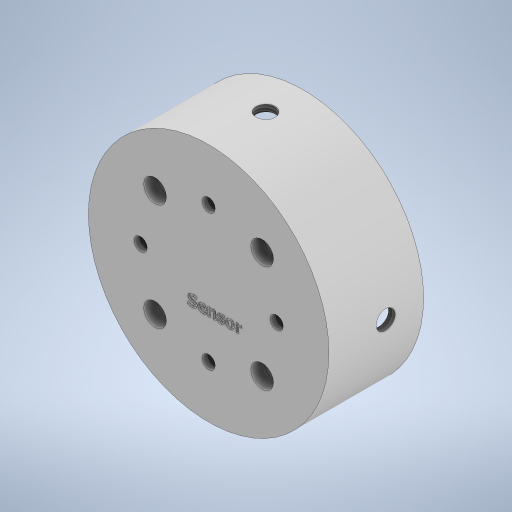
# Autodesk Inventor part: adaptor_sensor_spine
Saved by Autodesk Inventor 2024 (Build 280153000, 153)
## iProperties
Created: 2024-05-24
Part Number: adaptor_sensor_spine
Material: Generic
Document SubType Name: Modeling
Designer: maint
Density: 1 g/cm^3
Appearance: Default
Author: maint
Autodesk Inventor part; units mm, degrees
ref_plane "YZ Plane" through (0, 0, 0) normal (1, 0, 0) x (0, 1, 0)
sketch "Sketch1" plane through (0, 0, 0) normal (0, 0, 1) x (1, 0, 0)
  line L0 (40, -40) -> (-40, -40)
  line L1 (-40, -40) -> (-40, 40)
  line L2 (-40, 40) -> (40, 40)
  line L3 (40, 40) -> (40, -40)
  line L4 (40, -40) -> (-40, 40) construction
  line L5 (-40, -40) -> (40, 40) construction
  circle A0 centre (0, 0) radius 63.5
  dimension "d0" = 80
  dimension "d72" = 127
  constraints: 12 end point, 2 midpoint, 2 parallel, 2 perpendicular, 1 centre point, 1 coincident, 1 horizontal
  measures "d0" distance of L1.end L2.end
  measures "d72" diameter of A0
extrude "Extrusion1" add sketch "Sketch1" along normal blind 10 contours L0 L1 L2 L3 | A0
sketch "Sketch2" plane through (0, 0, 0) normal (0, 0, -1) x (-1, 0, 0)
  arc A0 (40, 37) -> (37, 40) centre (37, 37) ccw
  line L0 (28.2843, -28.2843) -> (-28.2843, -28.2843)
  line L1 (-28.2843, -28.2843) -> (-28.2843, 28.2843)
  line L2 (-28.2843, 28.2843) -> (28.2843, 28.2843)
  line L3 (28.2843, 28.2843) -> (28.2843, -28.2843)
  line L4 (28.2843, -28.2843) -> (-28.2843, 28.2843) construction
  line L5 (-28.2843, -28.2843) -> (28.2843, 28.2843) construction
  circle A1 centre (-28.2843, 28.2843) radius 4.75
  circle A2 centre (28.2843, 28.2843) radius 4.75
  circle A3 centre (28.2843, -28.2843) radius 4.75
  circle A4 centre (-28.2843, -28.2843) radius 4.75
  circle A5 centre (0, 0) radius 40
  point P0 (39.1213, 39.1213)
  dimension "d63" = 12
  dimension "d129" = 80
  dimension "d33" = 9.5
  constraints: 12 end point, 5 centre point, 5 coincident, 3 equal radius, 3 point on circle, 2 midpoint, 2 parallel, 2 perpendicular, 1 horizontal, 3 other
  measures "d33" diameter of A2
hole "Hole3" at (28.2843, -28.2843, 0) at (28.2843, 28.2843, 0) at (-28.2843, 28.2843, 0) at (-28.2843, -28.2843, 0) direction (0, 0, 1) diameter 6.6 end through all
sketch "Sketch10" plane through (0, 0, 10) normal (0, 0, 1) x (1, 0, 0)
  circle A0 centre (28.2843, 28.2843) radius 3.3 projected
  circle A1 centre (28.2843, 28.2843) radius 6
  circle A2 centre (-28.2843, 28.2843) radius 3.3 projected
  circle A3 centre (-28.2843, 28.2843) radius 6
  circle A4 centre (0, 0) radius 40
  line L0 (28.2843, 28.2843) -> (-28.2843, 28.2843)
  line L1 (-28.2843, 28.2843) -> (-28.2843, -28.2843)
  line L2 (-28.2843, -28.2843) -> (28.2843, -28.2843)
  line L3 (28.2843, -28.2843) -> (28.2843, 28.2843)
  circle A5 centre (-28.2843, -28.2843) radius 3.3 projected
  circle A6 centre (-28.2843, -28.2843) radius 6
  circle A7 centre (28.2843, -28.2843) radius 6
  dimension "d63" = 12
  dimension "d127" = 80
  constraints: 8 end point, 5 centre point, 5 coincident, 3 equal radius, 2 parallel, 1 horizontal, 1 perpendicular
  measures "d63" diameter of A1
  measures "d127" diameter of A4
sketch "Sketch11" plane through (-1.9817, 2.6504, 0) normal (0, 0, -1) x (-1, 0, 0)
  line L0 (-12.9782, -14.2221) -> (9.0418, -14.2221) construction
  line L1 (9.0418, -14.2221) -> (9.0418, -6.8756) construction
  line L2 (9.0418, -6.8756) -> (-12.9782, -6.8756) construction
  line L3 (-12.9782, -6.8756) -> (-12.9782, -14.2221) construction
  spline S0 degree 2 poles (-10.4621, -20.5396) (-11.164, -20.5396) (-12.2219, -20.2677) (-12.6767, -20.07) knots 0 0 0 1 2 2 2
  line L4 (-12.6767, -20.07) -> (-12.6767, -18.6166)
  line L5 (-12.6767, -18.6166) -> (-12.5383, -18.6166)
  spline S1 degree 2 poles (-12.5383, -18.6166) (-12.0785, -19.0072) (-10.9762, -19.4273) (-10.4571, -19.4273) knots 0 0 0 1 2 2 2
  spline S2 degree 2 poles (-10.4571, -19.4273) (-10.3237, -19.4273) (-9.8936, -19.368) (-9.7651, -19.3087) knots 0 0 0 1 2 2 2
  spline S3 degree 2 poles (-9.7651, -19.3087) (-9.6069, -19.2395) (-9.3845, -18.9874) (-9.3845, -18.7847) knots 0 0 0 1 2 2 2
  spline S4 degree 2 poles (-9.3845, -18.7847) (-9.3845, -18.5524) (-9.7453, -18.2657) (-9.9925, -18.2014) knots 0 0 0 1 2 2 2
  spline S5 degree 2 poles (-9.9925, -18.2014) (-10.3039, -18.1174) (-11.0108, -17.974) (-11.3222, -17.8653) knots 0 0 0 1 2 2 2
  spline S6 degree 2 poles (-11.3222, -17.8653) (-12.0291, -17.6181) (-12.6421, -16.7728) (-12.6421, -16.1401) knots 0 0 0 1 2 2 2
  spline S7 degree 2 poles (-12.6421, -16.1401) (-12.6421, -15.2849) (-11.1937, -14.2221) (-10.1062, -14.2221) knots 0 0 0 1 2 2 2
  spline S8 degree 2 poles (-10.1062, -14.2221) (-9.5624, -14.2221) (-8.4848, -14.4445) (-8.0597, -14.6324) knots 0 0 0 1 2 2 2
  line L6 (-8.0597, -14.6324) -> (-8.0597, -16.0264)
  line L7 (-8.0597, -16.0264) -> (-8.1931, -16.0264)
  spline S9 degree 2 poles (-8.1931, -16.0264) (-8.5342, -15.7347) (-9.513, -15.3343) (-10.0271, -15.3343) knots 0 0 0 1 2 2 2
  spline S10 degree 2 poles (-10.0271, -15.3343) (-10.2298, -15.3343) (-10.5461, -15.3936) (-10.7241, -15.4727) knots 0 0 0 1 2 2 2
  spline S11 degree 2 poles (-10.7241, -15.4727) (-10.8674, -15.537) (-11.0751, -15.794) (-11.0751, -15.9522) knots 0 0 0 1 2 2 2
  spline S12 degree 2 poles (-11.0751, -15.9522) (-11.0751, -16.1895) (-10.7439, -16.4614) (-10.2693, -16.5701) knots 0 0 0 1 2 2 2
  spline S13 degree 2 poles (-10.2693, -16.5701) (-9.9628, -16.6393) (-9.3943, -16.7728) (-9.0681, -16.8865) knots 0 0 0 1 2 2 2
  spline S14 degree 2 poles (-9.0681, -16.8865) (-8.4353, -17.1188) (-7.8174, -17.89) (-7.8174, -18.5227) knots 0 0 0 1 2 2 2
  spline S15 degree 2 poles (-7.8174, -18.5227) (-7.8174, -19.4323) (-9.246, -20.5396) (-10.4621, -20.5396) knots 0 0 0 1 2 2 2
  spline S16 degree 2 poles (-2.3403, -16.2538) (-2.3403, -16.6789) (-2.6122, -17.45) (-2.8643, -17.7071) knots 0 0 0 1 2 2 2
  spline S17 degree 2 poles (-2.8643, -17.7071) (-3.0175, -17.8702) (-3.3932, -18.1371) (-3.6157, -18.2311) knots 0 0 0 1 2 2 2
  spline S18 degree 2 poles (-3.6157, -18.2311) (-3.843, -18.325) (-4.372, -18.4337) (-4.6982, -18.4337) knots 0 0 0 1 2 2 2
  line L8 (-4.6982, -18.4337) -> (-5.499, -18.4337)
  line L9 (-5.499, -18.4337) -> (-5.499, -20.4308)
  line L10 (-5.499, -20.4308) -> (-7.0315, -20.4308)
  line L11 (-7.0315, -20.4308) -> (-7.0315, -14.3308)
  line L12 (-7.0315, -14.3308) -> (-4.6636, -14.3308)
  spline S19 degree 2 poles (-4.6636, -14.3308) (-4.1396, -14.3308) (-3.3734, -14.5236) (-3.062, -14.7312) knots 0 0 0 1 2 2 2
  spline S20 degree 2 poles (-3.062, -14.7312) (-2.716, -14.9636) (-2.3403, -15.7248) (-2.3403, -16.2538) knots 0 0 0 1 2 2 2
  spline S21 degree 2 poles (-3.9122, -16.2933) (-3.9122, -16.0313) (-4.1594, -15.6606) (-4.3275, -15.5914) knots 0 0 0 1 2 2 2
  spline S22 degree 2 poles (-4.3275, -15.5914) (-4.545, -15.4974) (-4.9404, -15.4678) (-5.2815, -15.4678) knots 0 0 0 1 2 2 2
  line L13 (-5.2815, -15.4678) -> (-5.499, -15.4678)
  line L14 (-5.499, -15.4678) -> (-5.499, -17.2968)
  line L15 (-5.499, -17.2968) -> (-5.3903, -17.2968)
  spline S23 degree 2 poles (-5.3903, -17.2968) (-5.1777, -17.2968) (-4.7922, -17.2869) (-4.6488, -17.2622) knots 0 0 0 1 2 2 2
  spline S24 degree 2 poles (-4.6488, -17.2622) (-4.5252, -17.2424) (-4.2533, -17.1238) (-4.1792, -17.0496) knots 0 0 0 1 2 2 2
  spline S25 degree 2 poles (-4.1792, -17.0496) (-4.021, -16.9013) (-3.9122, -16.5701) (-3.9122, -16.2933) knots 0 0 0 1 2 2 2
  line L16 (1.5155, -20.4308) -> (-1.7669, -20.4308)
  line L17 (-1.7669, -20.4308) -> (-1.7669, -19.368)
  line L18 (-1.7669, -19.368) -> (-0.8919, -19.368)
  line L19 (-0.8919, -19.368) -> (-0.8919, -15.3936)
  line L20 (-0.8919, -15.3936) -> (-1.7669, -15.3936)
  line L21 (-1.7669, -15.3936) -> (-1.7669, -14.3308)
  line L22 (-1.7669, -14.3308) -> (1.5155, -14.3308)
  line L23 (1.5155, -14.3308) -> (1.5155, -15.3936)
  line L24 (1.5155, -15.3936) -> (0.6405, -15.3936)
  line L25 (0.6405, -15.3936) -> (0.6405, -19.368)
  line L26 (0.6405, -19.368) -> (1.5155, -19.368)
  line L27 (1.5155, -19.368) -> (1.5155, -20.4308)
  line L28 (7.7588, -20.4308) -> (6.2857, -20.4308)
  line L29 (6.2857, -20.4308) -> (3.9327, -16.1796)
  line L30 (3.9327, -16.1796) -> (3.9327, -20.4308)
  line L31 (3.9327, -20.4308) -> (2.5338, -20.4308)
  line L32 (2.5338, -20.4308) -> (2.5338, -14.3308)
  line L33 (2.5338, -14.3308) -> (4.4122, -14.3308)
  line L34 (4.4122, -14.3308) -> (6.3599, -17.8257)
  line L35 (6.3599, -17.8257) -> (6.3599, -14.3308)
  line L36 (6.3599, -14.3308) -> (7.7588, -14.3308)
  line L37 (7.7588, -14.3308) -> (7.7588, -20.4308)
  line L38 (8.9996, -20.4308) -> (8.9996, -14.3308)
  line L39 (8.9996, -14.3308) -> (13.1223, -14.3308)
  line L40 (13.1223, -14.3308) -> (13.1223, -15.4925)
  line L41 (13.1223, -15.4925) -> (10.5221, -15.4925)
  line L42 (10.5221, -15.4925) -> (10.5221, -16.5652)
  line L43 (10.5221, -16.5652) -> (12.9196, -16.5652)
  line L44 (12.9196, -16.5652) -> (12.9196, -17.7268)
  line L45 (12.9196, -17.7268) -> (10.5221, -17.7268)
  line L46 (10.5221, -17.7268) -> (10.5221, -19.2692)
  line L47 (10.5221, -19.2692) -> (13.1223, -19.2692)
  line L48 (13.1223, -19.2692) -> (13.1223, -20.4308)
  line L49 (13.1223, -20.4308) -> (8.9996, -20.4308)
  point P0 (0, 0)
  constraints: 2 other
extrude "Extrusion5" cut sketch "Sketch11" against normal blind 1
sketch "Sketch12" plane through (-4.4722, 1.3995, 10) normal (0, 0, 1) x (1, 0, 0)
  line L0 (-6.7643, -10.3972) -> (19.0988, -10.3972) construction
  line L1 (19.0988, -10.3972) -> (19.0988, -6.1489) construction
  line L2 (19.0988, -6.1489) -> (-6.7643, -6.1489) construction
  line L3 (-6.7643, -6.1489) -> (-6.7643, -10.3972) construction
  spline S0 degree 2 poles (-4.2481, -16.7147) (-4.9501, -16.7147) (-6.0079, -16.4428) (-6.4627, -16.2451) knots 0 0 0 1 2 2 2
  line L4 (-6.4627, -16.2451) -> (-6.4627, -14.7918)
  line L5 (-6.4627, -14.7918) -> (-6.3243, -14.7918)
  spline S1 degree 2 poles (-6.3243, -14.7918) (-5.8646, -15.1823) (-4.7622, -15.6025) (-4.2432, -15.6025) knots 0 0 0 1 2 2 2
  spline S2 degree 2 poles (-4.2432, -15.6025) (-4.1097, -15.6025) (-3.6797, -15.5432) (-3.5511, -15.4838) knots 0 0 0 1 2 2 2
  spline S3 degree 2 poles (-3.5511, -15.4838) (-3.3929, -15.4146) (-3.1705, -15.1625) (-3.1705, -14.9599) knots 0 0 0 1 2 2 2
  spline S4 degree 2 poles (-3.1705, -14.9599) (-3.1705, -14.7275) (-3.5314, -14.4408) (-3.7785, -14.3765) knots 0 0 0 1 2 2 2
  spline S5 degree 2 poles (-3.7785, -14.3765) (-4.0899, -14.2925) (-4.7968, -14.1492) (-5.1083, -14.0404) knots 0 0 0 1 2 2 2
  spline S6 degree 2 poles (-5.1083, -14.0404) (-5.8152, -13.7932) (-6.4281, -12.9479) (-6.4281, -12.3152) knots 0 0 0 1 2 2 2
  spline S7 degree 2 poles (-6.4281, -12.3152) (-6.4281, -11.46) (-4.9797, -10.3972) (-3.8922, -10.3972) knots 0 0 0 1 2 2 2
  spline S8 degree 2 poles (-3.8922, -10.3972) (-3.3485, -10.3972) (-2.2708, -10.6197) (-1.8457, -10.8075) knots 0 0 0 1 2 2 2
  line L6 (-1.8457, -10.8075) -> (-1.8457, -12.2015)
  line L7 (-1.8457, -12.2015) -> (-1.9792, -12.2015)
  spline S9 degree 2 poles (-1.9792, -12.2015) (-2.3203, -11.9099) (-3.299, -11.5094) (-3.8131, -11.5094) knots 0 0 0 1 2 2 2
  spline S10 degree 2 poles (-3.8131, -11.5094) (-4.0158, -11.5094) (-4.3322, -11.5688) (-4.5101, -11.6479) knots 0 0 0 1 2 2 2
  spline S11 degree 2 poles (-4.5101, -11.6479) (-4.6535, -11.7121) (-4.8611, -11.9692) (-4.8611, -12.1274) knots 0 0 0 1 2 2 2
  spline S12 degree 2 poles (-4.8611, -12.1274) (-4.8611, -12.3646) (-4.5299, -12.6365) (-4.0553, -12.7453) knots 0 0 0 1 2 2 2
  spline S13 degree 2 poles (-4.0553, -12.7453) (-3.7489, -12.8145) (-3.1804, -12.9479) (-2.8541, -13.0616) knots 0 0 0 1 2 2 2
  spline S14 degree 2 poles (-2.8541, -13.0616) (-2.2214, -13.294) (-1.6035, -14.0651) (-1.6035, -14.6979) knots 0 0 0 1 2 2 2
  spline S15 degree 2 poles (-1.6035, -14.6979) (-1.6035, -15.6074) (-3.0321, -16.7147) (-4.2481, -16.7147) knots 0 0 0 1 2 2 2
  spline S16 degree 2 poles (1.4564, -16.7295) (0.1514, -16.7295) (-1.2377, -15.4838) (-1.2377, -14.3321) knots 0 0 0 1 2 2 2
  spline S17 degree 2 poles (-1.2377, -14.3321) (-1.2377, -13.205) (0.0575, -11.8604) (1.2241, -11.8604) knots 0 0 0 1 2 2 2
  spline S18 degree 2 poles (1.2241, -11.8604) (2.277, -11.8604) (3.3447, -13.0023) (3.3447, -14.0602) knots 0 0 0 1 2 2 2
  line L8 (3.3447, -14.0602) -> (3.3447, -14.5792)
  line L9 (3.3447, -14.5792) -> (0.1959, -14.5792)
  spline S19 degree 2 poles (0.1959, -14.5792) (0.2156, -14.9005) (0.448, -15.3257) (0.6358, -15.4542) knots 0 0 0 1 2 2 2
  spline S20 degree 2 poles (0.6358, -15.4542) (0.8187, -15.5827) (1.3131, -15.6915) (1.6047, -15.6915) knots 0 0 0 1 2 2 2
  spline S21 degree 2 poles (1.6047, -15.6915) (1.8519, -15.6915) (2.3363, -15.5827) (2.539, -15.4888) knots 0 0 0 1 2 2 2
  spline S22 degree 2 poles (2.539, -15.4888) (2.7169, -15.4146) (3.0135, -15.2317) (3.1075, -15.1625) knots 0 0 0 1 2 2 2
  line L10 (3.1075, -15.1625) -> (3.2607, -15.1625)
  line L11 (3.2607, -15.1625) -> (3.2607, -16.3489)
  spline S23 degree 2 poles (3.2607, -16.3489) (3.0827, -16.4181) (2.796, -16.5368) (2.539, -16.5961) knots 0 0 0 1 2 2 2
  spline S24 degree 2 poles (2.539, -16.5961) (2.3066, -16.6603) (1.8123, -16.7295) (1.4564, -16.7295) knots 0 0 0 1 2 2 2
  spline S25 degree 2 poles (1.931, -13.7141) (1.9211, -13.2594) (1.5207, -12.7799) (1.1104, -12.7799) knots 0 0 0 1 2 2 2
  spline S26 degree 2 poles (1.1104, -12.7799) (0.6902, -12.7799) (0.2156, -13.2841) (0.1909, -13.7141) knots 0 0 0 1 2 2 2
  line L12 (0.1909, -13.7141) -> (1.931, -13.7141)
  line L13 (8.3869, -16.606) -> (6.9434, -16.606)
  line L14 (6.9434, -16.606) -> (6.9434, -14.3271)
  spline S27 degree 2 poles (6.9434, -14.3271) (6.9434, -14.0453) (6.8989, -13.4917) (6.8396, -13.3632) knots 0 0 0 1 2 2 2
  spline S28 degree 2 poles (6.8396, -13.3632) (6.7655, -13.205) (6.4887, -13.0715) (6.2514, -13.0715) knots 0 0 0 1 2 2 2
  spline S29 degree 2 poles (6.2514, -13.0715) (6.0784, -13.0715) (5.7175, -13.205) (5.5148, -13.3483) knots 0 0 0 1 2 2 2
  line L15 (5.5148, -13.3483) -> (5.5148, -16.606)
  line L16 (5.5148, -16.606) -> (4.0813, -16.606)
  line L17 (4.0813, -16.606) -> (4.0813, -12.0038)
  line L18 (4.0813, -12.0038) -> (5.5148, -12.0038)
  line L19 (5.5148, -12.0038) -> (5.5148, -12.5129)
  spline S30 degree 2 poles (5.5148, -12.5129) (5.8658, -12.2163) (6.5331, -11.8802) (6.9385, -11.8802) knots 0 0 0 1 2 2 2
  spline S31 degree 2 poles (6.9385, -11.8802) (7.6404, -11.8802) (8.3869, -12.77) (8.3869, -13.6103) knots 0 0 0 1 2 2 2
  line L20 (8.3869, -13.6103) -> (8.3869, -16.606)
  spline S32 degree 2 poles (10.8486, -16.7295) (10.3444, -16.7295) (9.4398, -16.5071) (9.1432, -16.3588) knots 0 0 0 1 2 2 2
  line L21 (9.1432, -16.3588) -> (9.1432, -15.1477)
  line L22 (9.1432, -15.1477) -> (9.2618, -15.1477)
  spline S33 degree 2 poles (9.2618, -15.1477) (9.3656, -15.2268) (9.6276, -15.4146) (9.86, -15.5184) knots 0 0 0 1 2 2 2
  spline S34 degree 2 poles (9.86, -15.5184) (10.0626, -15.6124) (10.5619, -15.7458) (10.8585, -15.7458) knots 0 0 0 1 2 2 2
  spline S35 degree 2 poles (10.8585, -15.7458) (11.1601, -15.7458) (11.6247, -15.558) (11.6247, -15.3553) knots 0 0 0 1 2 2 2
  spline S36 degree 2 poles (11.6247, -15.3553) (11.6247, -15.1971) (11.4122, -15.0291) (11.1057, -14.9599) knots 0 0 0 1 2 2 2
  spline S37 degree 2 poles (11.1057, -14.9599) (10.9425, -14.9154) (10.4433, -14.8214) (10.2505, -14.7621) knots 0 0 0 1 2 2 2
  spline S38 degree 2 poles (10.2505, -14.7621) (9.7067, -14.594) (9.163, -13.9366) (9.163, -13.3978) knots 0 0 0 1 2 2 2
  spline S39 degree 2 poles (9.163, -13.3978) (9.163, -13.0913) (9.4447, -12.5475) (9.7216, -12.335) knots 0 0 0 1 2 2 2
  spline S40 degree 2 poles (9.7216, -12.335) (9.9934, -12.1274) (10.7992, -11.8802) (11.3084, -11.8802) knots 0 0 0 1 2 2 2
  spline S41 degree 2 poles (11.3084, -11.8802) (11.7928, -11.8802) (12.6035, -12.073) (12.8803, -12.2064) knots 0 0 0 1 2 2 2
  line L23 (12.8803, -12.2064) -> (12.8803, -13.3731)
  line L24 (12.8803, -13.3731) -> (12.7666, -13.3731)
  spline S42 degree 2 poles (12.7666, -13.3731) (12.6925, -13.3137) (12.3712, -13.121) (12.2229, -13.0517) knots 0 0 0 1 2 2 2
  spline S43 degree 2 poles (12.2229, -13.0517) (12.04, -12.9727) (11.5951, -12.8639) (11.3627, -12.8639) knots 0 0 0 1 2 2 2
  spline S44 degree 2 poles (11.3627, -12.8639) (11.0513, -12.8639) (10.6212, -13.0765) (10.6212, -13.2495) knots 0 0 0 1 2 2 2
  spline S45 degree 2 poles (10.6212, -13.2495) (10.6212, -13.4077) (10.8338, -13.5856) (11.1897, -13.6746) knots 0 0 0 1 2 2 2
  spline S46 degree 2 poles (11.1897, -13.6746) (11.3726, -13.7191) (11.8521, -13.8031) (12.0746, -13.8773) knots 0 0 0 1 2 2 2
  spline S47 degree 2 poles (12.0746, -13.8773) (12.5689, -14.0355) (13.083, -14.6534) (13.083, -15.1675) knots 0 0 0 1 2 2 2
  spline S48 degree 2 poles (13.083, -15.1675) (13.083, -15.4888) (12.7814, -16.077) (12.4997, -16.2748) knots 0 0 0 1 2 2 2
  spline S49 degree 2 poles (12.4997, -16.2748) (12.208, -16.4923) (11.4072, -16.7295) (10.8486, -16.7295) knots 0 0 0 1 2 2 2
  spline S50 degree 2 poles (18.1795, -14.3073) (18.1795, -15.4443) (16.9387, -16.7493) (15.8067, -16.7493) knots 0 0 0 1 2 2 2
  spline S51 degree 2 poles (15.8067, -16.7493) (14.6797, -16.7493) (13.429, -15.4443) (13.429, -14.3073) knots 0 0 0 1 2 2 2
  spline S52 degree 2 poles (13.429, -14.3073) (13.429, -13.1605) (14.6797, -11.8604) (15.8067, -11.8604) knots 0 0 0 1 2 2 2
  spline S53 degree 2 poles (15.8067, -11.8604) (16.9338, -11.8604) (18.1795, -13.1654) (18.1795, -14.3073) knots 0 0 0 1 2 2 2
  spline S54 degree 2 poles (16.7113, -14.3172) (16.7113, -13.9069) (16.5779, -13.3582) (16.4592, -13.1951) knots 0 0 0 1 2 2 2
  spline S55 degree 2 poles (16.4592, -13.1951) (16.3307, -13.0221) (16.0094, -12.8886) (15.8067, -12.8886) knots 0 0 0 1 2 2 2
  spline S56 degree 2 poles (15.8067, -12.8886) (15.609, -12.8886) (15.2976, -13.0073) (15.169, -13.1753) knots 0 0 0 1 2 2 2
  spline S57 degree 2 poles (15.169, -13.1753) (15.0455, -13.3335) (14.8972, -13.8921) (14.8972, -14.3172) knots 0 0 0 1 2 2 2
  spline S58 degree 2 poles (14.8972, -14.3172) (14.8972, -14.7374) (15.0356, -15.2564) (15.1493, -15.4146) knots 0 0 0 1 2 2 2
  spline S59 degree 2 poles (15.1493, -15.4146) (15.263, -15.5728) (15.609, -15.7211) (15.8166, -15.7211) knots 0 0 0 1 2 2 2
  spline S60 degree 2 poles (15.8166, -15.7211) (15.9896, -15.7211) (16.3455, -15.5728) (16.4543, -15.4245) knots 0 0 0 1 2 2 2
  spline S61 degree 2 poles (16.4543, -15.4245) (16.5779, -15.2515) (16.7113, -14.7522) (16.7113, -14.3172) knots 0 0 0 1 2 2 2
  line L25 (22.0303, -13.3632) -> (21.9117, -13.3632)
  spline S62 degree 2 poles (21.9117, -13.3632) (21.8276, -13.3335) (21.5162, -13.3039) (21.3284, -13.3039) knots 0 0 0 1 2 2 2
  spline S63 degree 2 poles (21.3284, -13.3039) (21.1059, -13.3039) (20.6066, -13.4373) (20.3743, -13.5263) knots 0 0 0 1 2 2 2
  line L26 (20.3743, -13.5263) -> (20.3743, -16.606)
  line L27 (20.3743, -16.606) -> (18.9408, -16.606)
  line L28 (18.9408, -16.606) -> (18.9408, -12.0038)
  line L29 (18.9408, -12.0038) -> (20.3743, -12.0038)
  line L30 (20.3743, -12.0038) -> (20.3743, -12.6662)
  spline S64 degree 2 poles (20.3743, -12.6662) (20.4732, -12.5772) (20.8192, -12.3004) (20.9626, -12.2163) knots 0 0 0 1 2 2 2
  spline S65 degree 2 poles (20.9626, -12.2163) (21.1207, -12.1224) (21.536, -11.9889) (21.7189, -11.9889) knots 0 0 0 1 2 2 2
  spline S66 degree 2 poles (21.7189, -11.9889) (21.7881, -11.9889) (21.9611, -11.9988) (22.0303, -12.0038) knots 0 0 0 1 2 2 2
  line L31 (22.0303, -12.0038) -> (22.0303, -13.3632)
  point P0 (0, 0)
  constraints: 2 other
extrude "Extrusion6" cut sketch "Sketch12" against normal blind 1
sketch "Sketch13" plane through (-11.7041, 34.1674, 0) normal (0, 0, -1) x (-1, 0, 0)
  line L0 (-1.7664, -61.241) -> (-17.5943, -76.9041) construction
  line L1 (-17.5943, -76.9041) -> (-22.3671, -72.081) construction
  line L2 (-22.3671, -72.081) -> (-6.5391, -56.4179) construction
  line L3 (-6.5391, -56.4179) -> (-1.7664, -61.241) construction
  line L4 (-5.7167, -57.8268) -> (-9.8926, -61.9592) construction
  line L5 (-9.8926, -61.9592) -> (-35.8899, -35.6882) construction
  line L6 (-35.8899, -35.6882) -> (-31.714, -31.5558) construction
  line L7 (-31.714, -31.5558) -> (-5.7167, -57.8268) construction
  line L8 (-5.3015, -58.7064) -> (-0.2981, -58.7064) construction
  line L9 (-0.2981, -58.7064) -> (-0.2981, -61.8764) construction
  line L10 (-0.2981, -61.8764) -> (-5.3015, -61.8764) construction
  line L11 (-5.3015, -61.8764) -> (-5.3015, -58.7064) construction
  line L12 (-17.522, -55.7631) -> (-14.084, -55.7631) construction
  line L13 (-14.084, -55.7631) -> (-14.084, -61.3066) construction
  line L14 (-14.084, -61.3066) -> (-17.522, -61.3066) construction
  line L15 (-17.522, -61.3066) -> (-17.522, -55.7631) construction
  line L16 (-7.756, -62.0484) -> (-6.5724, -62.0437)
  line L17 (-6.5724, -62.0437) -> (-6.5566, -57.4699)
  line L18 (-6.5566, -57.4699) -> (-6.0327, -57.4591)
  line L19 (-6.0327, -57.4591) -> (-6.0594, -62.0437)
  line L20 (-6.0594, -62.0437) -> (-4.8922, -62.0552)
  line L21 (-4.8922, -62.0552) -> (-6.3372, -65.8452)
  line L22 (-6.3372, -65.8452) -> (-7.756, -62.0484)
  line L23 (-10.7, -55.9696) -> (-10.6954, -57.1531)
  line L24 (-10.6954, -57.1531) -> (-6.1216, -57.1689)
  line L25 (-6.1216, -57.1689) -> (-6.1107, -57.6929)
  line L26 (-6.1107, -57.6929) -> (-10.6953, -57.6661)
  line L27 (-10.6953, -57.6661) -> (-10.7069, -58.8333)
  line L28 (-10.7069, -58.8333) -> (-14.4968, -57.3884)
  line L29 (-14.4968, -57.3884) -> (-10.7, -55.9696)
  line L30 (-14.5113, -58.9331) -> (-15.4309, -58.9331)
  line L31 (-15.4309, -58.9331) -> (-16.0423, -57.9235)
  line L32 (-16.0423, -57.9235) -> (-16.6666, -58.9331)
  line L33 (-16.6666, -58.9331) -> (-17.5477, -58.9331)
  line L34 (-17.5477, -58.9331) -> (-16.5176, -57.3378)
  line L35 (-16.5176, -57.3378) -> (-17.5066, -55.7631)
  line L36 (-17.5066, -55.7631) -> (-16.5869, -55.7631)
  line L37 (-16.5869, -55.7631) -> (-16.0141, -56.7213)
  line L38 (-16.0141, -56.7213) -> (-15.4258, -55.7631)
  line L39 (-15.4258, -55.7631) -> (-14.5447, -55.7631)
  line L40 (-14.5447, -55.7631) -> (-15.5388, -57.3044)
  line L41 (-15.5388, -57.3044) -> (-14.5113, -58.9331)
  line L42 (-2.337, -58.7064) -> (-3.4313, -60.5534)
  line L43 (-3.4313, -60.5534) -> (-3.4313, -61.8764)
  line L44 (-3.4313, -61.8764) -> (-4.2277, -61.8764)
  line L45 (-4.2277, -61.8764) -> (-4.2277, -60.592)
  line L46 (-4.2277, -60.592) -> (-5.34, -58.7064)
  line L47 (-5.34, -58.7064) -> (-4.4332, -58.7064)
  line L48 (-4.4332, -58.7064) -> (-3.8141, -59.8367)
  line L49 (-3.8141, -59.8367) -> (-3.2155, -58.7064)
  line L50 (-3.2155, -58.7064) -> (-2.337, -58.7064)
  point P0 (0, 0)
  constraints: 8 other
extrude "Extrusion7" cut sketch "Sketch13" against normal blind 1
sketch "Sketch14" plane through (0, 0, 0) normal (0, 0, -1) x (-1, 0, 0)
  circle A0 centre (0, 0) radius 3.5 projected
  circle A1 centre (0, 0) radius 60
  circle A2 centre (-0.3746, -0.3656) radius 8.5 projected
  circle A3 centre (0, 0) radius 63.5
  circle A4 centre (0, 0) radius 63.5 projected
  dimension "d84" = 120
  dimension "d89" = 127
  constraints: 2 centre point, 2 coincident, 1 concentric
  measures "d84" diameter of A1
  measures "d89" diameter of A3
extrude "Extrusion8" add sketch "Sketch14" along normal blind 40 contours A3
sketch "Sketch17" plane through (0, 0, 0) normal (0, 0, -1) x (-1, 0, 0)
  line L0 (0, -35.9156) -> (-35.9156, 0)
  line L1 (-35.9156, 0) -> (0, 35.9156)
  line L2 (0, 35.9156) -> (35.9156, 0)
  line L3 (35.9156, 0) -> (0, -35.9156)
  line L4 (0, -35.9156) -> (0, 35.9156) construction
  line L5 (-35.9156, 0) -> (35.9156, 0) construction
  line L6 (0, 35.9156) -> (0, -35.9156)
  line L7 (-35.9156, 0) -> (35.9156, 0)
  circle A0 centre (0, 35.9156) radius 3.5
  circle A1 centre (-35.9156, 0) radius 3.5
  circle A2 centre (0, -35.9156) radius 3.5
  circle A3 centre (35.9156, 0) radius 3.5
  circle A4 centre (0, 35.9156) radius 6
  circle A5 centre (-35.9156, 0) radius 6
  circle A6 centre (0, -35.9156) radius 6
  circle A7 centre (42.7164, -0.0489) radius 6
  point P0 (0, 0)
  dimension "d91" = 71.8312
  dimension "d92" = 7
  dimension "d93" = 12
  constraints: 16 end point, 8 centre point, 7 coincident, 6 equal radius, 3 equal length, 2 midpoint, 2 perpendicular, 1 vertical
  measures "d91" distance of L0.start L1.end
  measures "d92" diameter of A0
  measures "d93" diameter of A4
extrude "Extrusion9" cut sketch "Sketch17" against normal blind 10 contours L3 A2 L0 | L6 A2 L3 | L0 A2 L6 | A3 L7 L3 | L3 L2 A3 A7 | A1 L1 L0 | L0 L7 A1 | L7 A3 L2 | A7 A3 | L1 A1 L7 | A0 L1 L6 | L6 L2 A0 | A0 L2 L1 picked at (37.6395, -0.004)
sketch "Sketch18" plane through (0, 0, 0) normal (0, 0, -1) x (-1, 0, 0)
  circle A0 centre (0, 35.9156) radius 3.5 projected
  circle A1 centre (0, 35.9156) radius 6
  line L0 (0.0779, 73.9296) -> (0.0779, -51.2778)
  line L1 (-76.1216, -0.0489) -> (86.0637, -0.0489)
  circle A2 centre (0, -36.0134) radius 6
  circle A3 centre (35.9156, 0) radius 3.5 projected
  circle A4 centre (35.9156, 0) radius 6
  circle A5 centre (-35.7598, 0) radius 6
  point P0 (0, 0)
  dimension "d96" = 12
  constraints: 4 centre point, 4 end point, 2 coincident, 2 symmetric about line, 1 equal radius, 1 horizontal, 1 vertical, 2 other
  measures "d96" diameter of A1
extrude "Extrusion10" cut sketch "Sketch18" against normal blind 7
ref_plane "Work Plane2" through (-63.5, 0, 0) normal (-1, 0, 0) x (0, 0, 1)
ref_plane "Work Plane3" through (0, 63.5, 0) normal (0, -1, 0) x (1, 0, 0)
sketch "Sketch21" plane through (-63.5, 0, 0) normal (-1, 0, 0) x (0, 0, 1)
  circle A0 centre (-20, 0) radius 5
  point P0 (0, 0)
  dimension "d104" = 20
  dimension "d105" = 10
  constraints: 1 centre point
  measures "d104" distance of point (0, 0) A0.centre
  measures "d105" diameter of A0
sketch "Sketch22" plane through (0, 63.5, 0) normal (0, -1, 0) x (1, 0, 0)
  circle A0 centre (0, -20) radius 5
  point P0 (0, 0)
  dimension "d101" = 10
  dimension "d106" = 20
  constraints: 1 centre point
  measures "d101" diameter of A0
  measures "d106" distance of point (0, 0) A0.centre
hole "Hole7" at (0, 63.5, -20) direction (0, -1, 0) diameter 10 depth 150
thread "Thread1" size "M10x1.5" class "6H" standard "ISO Metric profile" full length
extrude "Extrusion13" cut sketch "Sketch21" against normal blind 150
thread "Thread2" size "M10x1.5" class "6H" standard "ISO Metric profile" full length
extrude "Extrusion14" cut sketch "Sketch10" against normal blind 7 contours A0 A4 | A0 A4 A1 | A4 L0 A0 | A0 L0 A1 A4 | A4 A1 L3 A0 | A0 L3 A4 | L0 L3 A0 | A0 L3 A1 L0 | A4 A2 A3 | A3 L0 A2 A4 | A3 L1 A2 L0 | A4 A2 L1 A3 | A4 A2 | A2 L0 A4 | A7 A4 L3 | L3 L2 A7 | A7 A4 | A2 L1 L0 | A4 L1 A2 | A6 L1 A5 A4 | A4 A5 A6 | A4 A7 L2 | A6 L2 A5 L1 | A5 L1 A4 | A4 A5 | A4 A5 L2 A6 | A5 L2 L1 | L2 A5 A4
body "Solid1"
